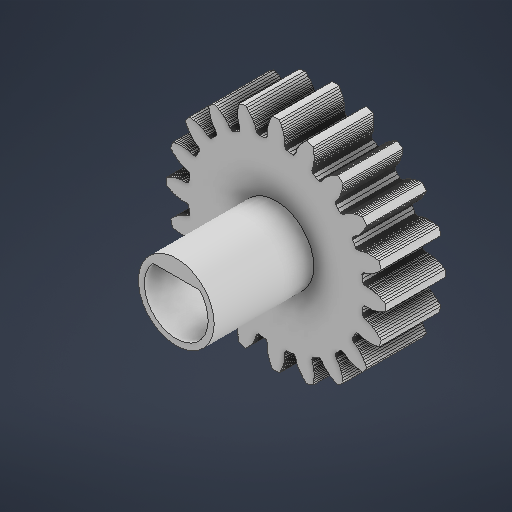
# Autodesk Inventor part: EngranajeMotor
Saved by Autodesk Inventor 2027 (Build 310192060, 192F)
## iProperties
Created: 2026-08-09
Part Number: EngranajeMotor
Material: Generic
Document SubType Name: Modeling
Designer: Administrator
Density: 1 g/cm^3
Appearance: Default
Author: Administrator
Autodesk Inventor part; units mm, degrees
(part 1 of 3)
ref_plane "YZ Plane" through (0, 0, 0) normal (1, 0, 0) x (0, 1, 0)
ref_plane "XZ Plane" through (0, 0, 0) normal (0, 1, 0) x (-1, 0, 0)
ref_plane "XY Plane" through (0, 0, 0) normal (0, 0, 1) x (1, 0, 0)
sketch "Sketch2" plane through (0, 0, 0) normal (0, 0, 1) x (1, 0, 0)
  arc A0 (-1.118, 1) -> (1.118, 1) centre (0, 0) ccw
  arc A1 (-1.118, 1) -> (1.118, 1) centre (0, 0) ccw
  line L0 (0, -0.275) -> (0, 0.275)
  line L1 (-0.275, 0) -> (0.275, 0)
  line L2 (0, -0.275) -> (0, 0.275)
  line L3 (-0.275, 0) -> (0.275, 0)
  line L4 (0, 1) -> (-1.118, 1)
  line L5 (0, 1) -> (1.118, 1)
  line L6 (5.0569, 1.3152) -> (4.9868, 1.2577)
  line L7 (4.9868, 1.2577) -> (4.9194, 1.207)
  line L8 (4.9194, 1.207) -> (4.8581, 1.1647)
  line L9 (4.8581, 1.1647) -> (4.8009, 1.1288)
  line L10 (4.8009, 1.1288) -> (4.75, 1.0997)
  line L11 (4.75, 1.0997) -> (4.7061, 1.0769)
  line L12 (4.7061, 1.0769) -> (4.6364, 1.046)
  line L13 (4.6364, 1.046) -> (4.5924, 1.0307)
  line L14 (4.5924, 1.0307) -> (4.5075, 1.0081)
  line L15 (4.5075, 1.0081) -> (4.4514, 0.9867)
  line L16 (4.4514, 0.9867) -> (4.427, 0.9751)
  line L17 (4.427, 0.9751) -> (4.4051, 0.9628)
  line L18 (4.4051, 0.9628) -> (4.3856, 0.9502)
  line L19 (4.3856, 0.9502) -> (4.3686, 0.9372)
  line L20 (4.3686, 0.9372) -> (4.354, 0.9239)
  line L21 (4.354, 0.9239) -> (4.3419, 0.9105)
  line L22 (4.3419, 0.9105) -> (4.3323, 0.897)
  line L23 (4.3323, 0.897) -> (4.3252, 0.8836)
  line L24 (4.3252, 0.8836) -> (4.3205, 0.8703)
  line L25 (4.3205, 0.8703) -> (4.3182, 0.8572)
  line L26 (4.3182, 0.8572) -> (4.3194, 0.8383)
  line L27 (4.3194, 0.8383) -> (4.3458, 0.6883)
  line L28 (4.3458, 0.6883) -> (4.3671, 0.5375)
  line L29 (4.3671, 0.5375) -> (4.3718, 0.5191)
  line L30 (4.3718, 0.5191) -> (4.378, 0.5074)
  line L31 (4.378, 0.5074) -> (4.3865, 0.4962)
  line L32 (4.3865, 0.4962) -> (4.3975, 0.4856)
  line L33 (4.3975, 0.4856) -> (4.4108, 0.4758)
  line L34 (4.4108, 0.4758) -> (4.4264, 0.4668)
  line L35 (4.4264, 0.4668) -> (4.4444, 0.4587)
  line L36 (4.4444, 0.4587) -> (4.4646, 0.4516)
  line L37 (4.4646, 0.4516) -> (4.487, 0.4455)
  line L38 (4.487, 0.4455) -> (4.5117, 0.4407)
  line L39 (4.5117, 0.4407) -> (4.5385, 0.4371)
  line L40 (4.5385, 0.4371) -> (4.5984, 0.4341)
  line L41 (4.5984, 0.4341) -> (4.6862, 0.4388)
  line L42 (4.6862, 0.4388) -> (4.7327, 0.438)
  line L43 (4.7327, 0.438) -> (4.8085, 0.43)
  line L44 (4.8085, 0.43) -> (4.8574, 0.422)
  line L45 (4.8574, 0.422) -> (4.9147, 0.41)
  line L46 (4.9147, 0.41) -> (4.9802, 0.3935)
  line L47 (4.9802, 0.3935) -> (5.0516, 0.3723)
  line L48 (5.0516, 0.3723) -> (5.1313, 0.3449)
  line L49 (5.1313, 0.3449) -> (5.2159, 0.3118)
  line L50 (5.2159, 0.3118) -> (5.3081, 0.2712)
  line L51 (5.3081, 0.2712) -> (5.4053, 0.2235)
  line L52 (5.4053, 0.2235) -> (5.4973, 0.1736)
  arc A2 (5.4973, -0.1736) -> (5.4973, 0.1736) centre (0, 0) ccw
  line L53 (5.4973, -0.1736) -> (5.4053, -0.2235)
  line L54 (5.4053, -0.2235) -> (5.3081, -0.2712)
  line L55 (5.3081, -0.2712) -> (5.2159, -0.3118)
  line L56 (5.2159, -0.3118) -> (5.1313, -0.3449)
  line L57 (5.1313, -0.3449) -> (5.0516, -0.3723)
  line L58 (5.0516, -0.3723) -> (4.9802, -0.3935)
  line L59 (4.9802, -0.3935) -> (4.9147, -0.41)
  line L60 (4.9147, -0.41) -> (4.8574, -0.422)
  line L61 (4.8574, -0.422) -> (4.8085, -0.43)
  line L62 (4.8085, -0.43) -> (4.7327, -0.438)
  line L63 (4.7327, -0.438) -> (4.6862, -0.4388)
  line L64 (4.6862, -0.4388) -> (4.5984, -0.4341)
  line L65 (4.5984, -0.4341) -> (4.5385, -0.4371)
  line L66 (4.5385, -0.4371) -> (4.5117, -0.4407)
  line L67 (4.5117, -0.4407) -> (4.487, -0.4455)
  line L68 (4.487, -0.4455) -> (4.4646, -0.4516)
  line L69 (4.4646, -0.4516) -> (4.4444, -0.4587)
  line L70 (4.4444, -0.4587) -> (4.4264, -0.4668)
  line L71 (4.4264, -0.4668) -> (4.4108, -0.4758)
  line L72 (4.4108, -0.4758) -> (4.3975, -0.4856)
  line L73 (4.3975, -0.4856) -> (4.3865, -0.4962)
  line L74 (4.3865, -0.4962) -> (4.378, -0.5074)
  line L75 (4.378, -0.5074) -> (4.3718, -0.5191)
  line L76 (4.3718, -0.5191) -> (4.3671, -0.5375)
  line L77 (4.3671, -0.5375) -> (4.3458, -0.6883)
  line L78 (4.3458, -0.6883) -> (4.3194, -0.8383)
  line L79 (4.3194, -0.8383) -> (4.3182, -0.8572)
  line L80 (4.3182, -0.8572) -> (4.3205, -0.8703)
  line L81 (4.3205, -0.8703) -> (4.3252, -0.8836)
  line L82 (4.3252, -0.8836) -> (4.3323, -0.897)
  line L83 (4.3323, -0.897) -> (4.3419, -0.9105)
  line L84 (4.3419, -0.9105) -> (4.354, -0.9239)
  line L85 (4.354, -0.9239) -> (4.3686, -0.9372)
  line L86 (4.3686, -0.9372) -> (4.3856, -0.9502)
  line L87 (4.3856, -0.9502) -> (4.4051, -0.9628)
  line L88 (4.4051, -0.9628) -> (4.427, -0.9751)
  line L89 (4.427, -0.9751) -> (4.4514, -0.9867)
  line L90 (4.4514, -0.9867) -> (4.5075, -1.0081)
  line L91 (4.5075, -1.0081) -> (4.5924, -1.0307)
  line L92 (4.5924, -1.0307) -> (4.6364, -1.046)
  line L93 (4.6364, -1.046) -> (4.7061, -1.0769)
  line L94 (4.7061, -1.0769) -> (4.75, -1.0997)
  line L95 (4.75, -1.0997) -> (4.8009, -1.1288)
  line L96 (4.8009, -1.1288) -> (4.8581, -1.1647)
  line L97 (4.8581, -1.1647) -> (4.9194, -1.207)
  line L98 (4.9194, -1.207) -> (4.9868, -1.2577)
  line L99 (4.9868, -1.2577) -> (5.0569, -1.3152)
  line L100 (5.0569, -1.3152) -> (5.1322, -1.3823)
  line L101 (5.1322, -1.3823) -> (5.2098, -1.4578)
  line L102 (5.2098, -1.4578) -> (5.2818, -1.5336)
  arc A3 (5.1745, -1.8639) -> (5.2818, -1.5336) centre (0, 0) ccw
  line L103 (5.1745, -1.8639) -> (5.0717, -1.8829)
  line L104 (5.0717, -1.8829) -> (4.9645, -1.8983)
  line L105 (4.9645, -1.8983) -> (4.8642, -1.9084)
  line L106 (4.8642, -1.9084) -> (4.7736, -1.9137)
  line L107 (4.7736, -1.9137) -> (4.6893, -1.9151)
  line L108 (4.6893, -1.9151) -> (4.6149, -1.9132)
  line L109 (4.6149, -1.9132) -> (4.5475, -1.9087)
  line L110 (4.5475, -1.9087) -> (4.4892, -1.9023)
  line L111 (4.4892, -1.9023) -> (4.4403, -1.8949)
  line L112 (4.4403, -1.8949) -> (4.3657, -1.879)
  line L113 (4.3657, -1.879) -> (4.3212, -1.8655)
  line L114 (4.3212, -1.8655) -> (4.2391, -1.8339)
  line L115 (4.2391, -1.8339) -> (4.1813, -1.8182)
  line L116 (4.1813, -1.8182) -> (4.1547, -1.8133)
  line L117 (4.1547, -1.8133) -> (4.1297, -1.8103)
  line L118 (4.1297, -1.8103) -> (4.1065, -1.8091)
  line L119 (4.1065, -1.8091) -> (4.0851, -1.8096)
  line L120 (4.0851, -1.8096) -> (4.0655, -1.8118)
  line L121 (4.0655, -1.8118) -> (4.0479, -1.8155)
  line L122 (4.0479, -1.8155) -> (4.0322, -1.8208)
  line L123 (4.0322, -1.8208) -> (4.0185, -1.8274)
  line L124 (4.0185, -1.8274) -> (4.0069, -1.8354)
  line L125 (4.0069, -1.8354) -> (3.9974, -1.8447)
  line L126 (3.9974, -1.8447) -> (3.9872, -1.8607)
  line L127 (3.9872, -1.8607) -> (3.9204, -1.9976)
  line L128 (3.9204, -1.9976) -> (3.8489, -2.1321)
  line L129 (3.8489, -2.1321) -> (3.842, -2.1497)
  line L130 (3.842, -2.1497) -> (3.8401, -2.1628)
  line L131 (3.8401, -2.1628) -> (3.8404, -2.1769)
  line L132 (3.8404, -2.1769) -> (3.8431, -2.1919)
  line L133 (3.8431, -2.1919) -> (3.8481, -2.2077)
  line L134 (3.8481, -2.2077) -> (3.8554, -2.2242)
  line L135 (3.8554, -2.2242) -> (3.8652, -2.2413)
  line L136 (3.8652, -2.2413) -> (3.8773, -2.2589)
  line L137 (3.8773, -2.2589) -> (3.892, -2.277)
  line L138 (3.892, -2.277) -> (3.9091, -2.2954)
  line L139 (3.9091, -2.2954) -> (3.9286, -2.314)
  line L140 (3.9286, -2.314) -> (3.9753, -2.3516)
  line L141 (3.9753, -2.3516) -> (4.0491, -2.3994)
  line L142 (4.0491, -2.3994) -> (4.0862, -2.4275)
  line L143 (4.0862, -2.4275) -> (4.1429, -2.4785)
  line L144 (4.1429, -2.4785) -> (4.1777, -2.5137)
  line L145 (4.1777, -2.5137) -> (4.2171, -2.5571)
  line L146 (4.2171, -2.5571) -> (4.2604, -2.609)
  line L147 (4.2604, -2.609) -> (4.3057, -2.6681)
  line L148 (4.3057, -2.6681) -> (4.3541, -2.7371)
  line L149 (4.3541, -2.7371) -> (4.403, -2.8135)
  line L150 (4.403, -2.8135) -> (4.4538, -2.9006)
  line L151 (4.4538, -2.9006) -> (4.5044, -2.9964)
  line L152 (4.5044, -2.9964) -> (4.5494, -3.0907)
  arc A4 (4.3453, -3.3717) -> (4.5494, -3.0907) centre (0, 0) ccw
  line L153 (4.3453, -3.3717) -> (4.2416, -3.358)
  line L154 (4.2416, -3.358) -> (4.1349, -3.3395)
  line L155 (4.1349, -3.3395) -> (4.0364, -3.3181)
  line L156 (4.0364, -3.3181) -> (3.9486, -3.2952)
  line L157 (3.9486, -3.2952) -> (3.868, -3.2704)
  line L158 (3.868, -3.2704) -> (3.7978, -3.2457)
  line L159 (3.7978, -3.2457) -> (3.7351, -3.2205)
  line L160 (3.7351, -3.2205) -> (3.6817, -3.1965)
  line L161 (3.6817, -3.1965) -> (3.6374, -3.1743)
  line L162 (3.6374, -3.1743) -> (3.5714, -3.1361)
  line L163 (3.5714, -3.1361) -> (3.5332, -3.1095)
  line L164 (3.5332, -3.1095) -> (3.465, -3.0541)
  line L165 (3.465, -3.0541) -> (3.4148, -3.0213)
  line L166 (3.4148, -3.0213) -> (3.391, -3.0084)
  line L167 (3.391, -3.0084) -> (3.3682, -2.9979)
  line L168 (3.3682, -2.9979) -> (3.3465, -2.9895)
  line L169 (3.3465, -2.9895) -> (3.326, -2.9834)
  line L170 (3.326, -2.9834) -> (3.3067, -2.9794)
  line L171 (3.3067, -2.9794) -> (3.2887, -2.9775)
  line L172 (3.2887, -2.9775) -> (3.2722, -2.9777)
  line L173 (3.2722, -2.9777) -> (3.2571, -2.9798)
  line L174 (3.2571, -2.9798) -> (3.2436, -2.9838)
  line L175 (3.2436, -2.9838) -> (3.2317, -2.9896)
  line L176 (3.2317, -2.9896) -> (3.2171, -3.0017)
  line L177 (3.2171, -3.0017) -> (3.1113, -3.1113)
  line L178 (3.1113, -3.1113) -> (3.0017, -3.2171)
  line L179 (3.0017, -3.2171) -> (2.9896, -3.2317)
  line L180 (2.9896, -3.2317) -> (2.9838, -3.2436)
  line L181 (2.9838, -3.2436) -> (2.9798, -3.2571)
  line L182 (2.9798, -3.2571) -> (2.9777, -3.2722)
  line L183 (2.9777, -3.2722) -> (2.9775, -3.2887)
  line L184 (2.9775, -3.2887) -> (2.9794, -3.3067)
  line L185 (2.9794, -3.3067) -> (2.9834, -3.326)
  line L186 (2.9834, -3.326) -> (2.9895, -3.3465)
  line L187 (2.9895, -3.3465) -> (2.9979, -3.3682)
  line L188 (2.9979, -3.3682) -> (3.0084, -3.391)
  line L189 (3.0084, -3.391) -> (3.0213, -3.4148)
  line L190 (3.0213, -3.4148) -> (3.0541, -3.465)
  line L191 (3.0541, -3.465) -> (3.1095, -3.5332)
  line L192 (3.1095, -3.5332) -> (3.1361, -3.5714)
  line L193 (3.1361, -3.5714) -> (3.1743, -3.6374)
  line L194 (3.1743, -3.6374) -> (3.1965, -3.6817)
  line L195 (3.1965, -3.6817) -> (3.2205, -3.7351)
  line L196 (3.2205, -3.7351) -> (3.2457, -3.7978)
  line L197 (3.2457, -3.7978) -> (3.2704, -3.868)
  line L198 (3.2704, -3.868) -> (3.2952, -3.9486)
  line L199 (3.2952, -3.9486) -> (3.3181, -4.0364)
  line L200 (3.3181, -4.0364) -> (3.3395, -4.1349)
  line L201 (3.3395, -4.1349) -> (3.358, -4.2416)
  line L202 (3.358, -4.2416) -> (3.3717, -4.3453)
  arc A5 (3.0907, -4.5494) -> (3.3717, -4.3453) centre (0, 0) ccw
  line L203 (3.0907, -4.5494) -> (2.9964, -4.5044)
  line L204 (2.9964, -4.5044) -> (2.9006, -4.4538)
  line L205 (2.9006, -4.4538) -> (2.8135, -4.403)
  line L206 (2.8135, -4.403) -> (2.7371, -4.3541)
  line L207 (2.7371, -4.3541) -> (2.6681, -4.3057)
  line L208 (2.6681, -4.3057) -> (2.609, -4.2604)
  line L209 (2.609, -4.2604) -> (2.5571, -4.2171)
  line L210 (2.5571, -4.2171) -> (2.5137, -4.1777)
  line L211 (2.5137, -4.1777) -> (2.4785, -4.1429)
  line L212 (2.4785, -4.1429) -> (2.4275, -4.0862)
  line L213 (2.4275, -4.0862) -> (2.3994, -4.0491)
  line L214 (2.3994, -4.0491) -> (2.3516, -3.9753)
  line L215 (2.3516, -3.9753) -> (2.314, -3.9286)
  line L216 (2.314, -3.9286) -> (2.2954, -3.9091)
  line L217 (2.2954, -3.9091) -> (2.277, -3.892)
  line L218 (2.277, -3.892) -> (2.2589, -3.8773)
  line L219 (2.2589, -3.8773) -> (2.2413, -3.8652)
  line L220 (2.2413, -3.8652) -> (2.2242, -3.8554)
  line L221 (2.2242, -3.8554) -> (2.2077, -3.8481)
  line L222 (2.2077, -3.8481) -> (2.1919, -3.8431)
  line L223 (2.1919, -3.8431) -> (2.1769, -3.8404)
  line L224 (2.1769, -3.8404) -> (2.1628, -3.8401)
  line L225 (2.1628, -3.8401) -> (2.1497, -3.842)
  line L226 (2.1497, -3.842) -> (2.1321, -3.8489)
  line L227 (2.1321, -3.8489) -> (1.9976, -3.9204)
  line L228 (1.9976, -3.9204) -> (1.8607, -3.9872)
  line L229 (1.8607, -3.9872) -> (1.8447, -3.9974)
  line L230 (1.8447, -3.9974) -> (1.8354, -4.0069)
  line L231 (1.8354, -4.0069) -> (1.8274, -4.0185)
  line L232 (1.8274, -4.0185) -> (1.8208, -4.0322)
  line L233 (1.8208, -4.0322) -> (1.8155, -4.0479)
  line L234 (1.8155, -4.0479) -> (1.8118, -4.0655)
  line L235 (1.8118, -4.0655) -> (1.8096, -4.0851)
  line L236 (1.8096, -4.0851) -> (1.8091, -4.1065)
  line L237 (1.8091, -4.1065) -> (1.8103, -4.1297)
  line L238 (1.8103, -4.1297) -> (1.8133, -4.1547)
  line L239 (1.8133, -4.1547) -> (1.8182, -4.1813)
  line L240 (1.8182, -4.1813) -> (1.8339, -4.2391)
  line L241 (1.8339, -4.2391) -> (1.8655, -4.3212)
  line L242 (1.8655, -4.3212) -> (1.879, -4.3657)
  line L243 (1.879, -4.3657) -> (1.8949, -4.4403)
  line L244 (1.8949, -4.4403) -> (1.9023, -4.4892)
  line L245 (1.9023, -4.4892) -> (1.9087, -4.5475)
  line L246 (1.9087, -4.5475) -> (1.9132, -4.6149)
  line L247 (1.9132, -4.6149) -> (1.9151, -4.6893)
  line L248 (1.9151, -4.6893) -> (1.9137, -4.7736)
  line L249 (1.9137, -4.7736) -> (1.9084, -4.8642)
  line L250 (1.9084, -4.8642) -> (1.8983, -4.9645)
  line L251 (1.8983, -4.9645) -> (1.8829, -5.0717)
  line L252 (1.8829, -5.0717) -> (1.8639, -5.1745)
  arc A6 (1.5336, -5.2818) -> (1.8639, -5.1745) centre (0, 0) ccw
  line L253 (1.5336, -5.2818) -> (1.4578, -5.2098)
  line L254 (1.4578, -5.2098) -> (1.3823, -5.1322)
  line L255 (1.3823, -5.1322) -> (1.3152, -5.0569)
  line L256 (1.3152, -5.0569) -> (1.2577, -4.9868)
  line L257 (1.2577, -4.9868) -> (1.207, -4.9194)
  line L258 (1.207, -4.9194) -> (1.1647, -4.8581)
  line L259 (1.1647, -4.8581) -> (1.1288, -4.8009)
  line L260 (1.1288, -4.8009) -> (1.0997, -4.75)
  line L261 (1.0997, -4.75) -> (1.0769, -4.7061)
  line L262 (1.0769, -4.7061) -> (1.046, -4.6364)
  line L263 (1.046, -4.6364) -> (1.0307, -4.5924)
  line L264 (1.0307, -4.5924) -> (1.0081, -4.5075)
  line L265 (1.0081, -4.5075) -> (0.9867, -4.4514)
  line L266 (0.9867, -4.4514) -> (0.9751, -4.427)
  line L267 (0.9751, -4.427) -> (0.9628, -4.4051)
  line L268 (0.9628, -4.4051) -> (0.9502, -4.3856)
  line L269 (0.9502, -4.3856) -> (0.9372, -4.3686)
  line L270 (0.9372, -4.3686) -> (0.9239, -4.354)
  line L271 (0.9239, -4.354) -> (0.9105, -4.3419)
  line L272 (0.9105, -4.3419) -> (0.897, -4.3323)
  line L273 (0.897, -4.3323) -> (0.8836, -4.3252)
  line L274 (0.8836, -4.3252) -> (0.8703, -4.3205)
  line L275 (0.8703, -4.3205) -> (0.8572, -4.3182)
  line L276 (0.8572, -4.3182) -> (0.8383, -4.3194)
  line L277 (0.8383, -4.3194) -> (0.6883, -4.3458)
  line L278 (0.6883, -4.3458) -> (0.5375, -4.3671)
  line L279 (0.5375, -4.3671) -> (0.5191, -4.3718)
  line L280 (0.5191, -4.3718) -> (0.5074, -4.378)
  line L281 (0.5074, -4.378) -> (0.4962, -4.3865)
  line L282 (0.4962, -4.3865) -> (0.4856, -4.3975)
  line L283 (0.4856, -4.3975) -> (0.4758, -4.4108)
  line L284 (0.4758, -4.4108) -> (0.4668, -4.4264)
  line L285 (0.4668, -4.4264) -> (0.4587, -4.4444)
  line L286 (0.4587, -4.4444) -> (0.4516, -4.4646)
  line L287 (0.4516, -4.4646) -> (0.4455, -4.487)
  line L288 (0.4455, -4.487) -> (0.4407, -4.5117)
  line L289 (0.4407, -4.5117) -> (0.4371, -4.5385)
  line L290 (0.4371, -4.5385) -> (0.4341, -4.5984)
  line L291 (0.4341, -4.5984) -> (0.4388, -4.6862)
  line L292 (0.4388, -4.6862) -> (0.438, -4.7327)
  line L293 (0.438, -4.7327) -> (0.43, -4.8085)
  line L294 (0.43, -4.8085) -> (0.422, -4.8574)
  line L295 (0.422, -4.8574) -> (0.41, -4.9147)
  line L296 (0.41, -4.9147) -> (0.3935, -4.9802)
  line L297 (0.3935, -4.9802) -> (0.3723, -5.0516)
  line L298 (0.3723, -5.0516) -> (0.3449, -5.1313)
  line L299 (0.3449, -5.1313) -> (0.3118, -5.2159)
  line L300 (0.3118, -5.2159) -> (0.2712, -5.3081)
  line L301 (0.2712, -5.3081) -> (0.2235, -5.4053)
  line L302 (0.2235, -5.4053) -> (0.1736, -5.4973)
  arc A7 (-0.1736, -5.4973) -> (0.1736, -5.4973) centre (0, 0) ccw
  line L303 (-0.1736, -5.4973) -> (-0.2235, -5.4053)
  line L304 (-0.2235, -5.4053) -> (-0.2712, -5.3081)
  line L305 (-0.2712, -5.3081) -> (-0.3118, -5.2159)
  line L306 (-0.3118, -5.2159) -> (-0.3449, -5.1313)
  line L307 (-0.3449, -5.1313) -> (-0.3723, -5.0516)
  line L308 (-0.3723, -5.0516) -> (-0.3935, -4.9802)
  line L309 (-0.3935, -4.9802) -> (-0.41, -4.9147)
  line L310 (-0.41, -4.9147) -> (-0.422, -4.8574)
  line L311 (-0.422, -4.8574) -> (-0.43, -4.8085)
  line L312 (-0.43, -4.8085) -> (-0.438, -4.7327)
  line L313 (-0.438, -4.7327) -> (-0.4388, -4.6862)
  line L314 (-0.4388, -4.6862) -> (-0.4341, -4.5984)
  line L315 (-0.4341, -4.5984) -> (-0.4371, -4.5385)
  line L316 (-0.4371, -4.5385) -> (-0.4407, -4.5117)
  line L317 (-0.4407, -4.5117) -> (-0.4455, -4.487)
  line L318 (-0.4455, -4.487) -> (-0.4516, -4.4646)
  line L319 (-0.4516, -4.4646) -> (-0.4587, -4.4444)
  line L320 (-0.4587, -4.4444) -> (-0.4668, -4.4264)
  line L321 (-0.4668, -4.4264) -> (-0.4758, -4.4108)
  line L322 (-0.4758, -4.4108) -> (-0.4856, -4.3975)
  line L323 (-0.4856, -4.3975) -> (-0.4962, -4.3865)
  line L324 (-0.4962, -4.3865) -> (-0.5074, -4.378)
  line L325 (-0.5074, -4.378) -> (-0.5191, -4.3718)
  line L326 (-0.5191, -4.3718) -> (-0.5375, -4.3671)
  line L327 (-0.5375, -4.3671) -> (-0.6883, -4.3458)
  line L328 (-0.6883, -4.3458) -> (-0.8383, -4.3194)
  line L329 (-0.8383, -4.3194) -> (-0.8572, -4.3182)
  line L330 (-0.8572, -4.3182) -> (-0.8703, -4.3205)
  line L331 (-0.8703, -4.3205) -> (-0.8836, -4.3252)
  line L332 (-0.8836, -4.3252) -> (-0.897, -4.3323)
  line L333 (-0.897, -4.3323) -> (-0.9105, -4.3419)
  line L334 (-0.9105, -4.3419) -> (-0.9239, -4.354)
  line L335 (-0.9239, -4.354) -> (-0.9372, -4.3686)
  line L336 (-0.9372, -4.3686) -> (-0.9502, -4.3856)
  line L337 (-0.9502, -4.3856) -> (-0.9628, -4.4051)
  line L338 (-0.9628, -4.4051) -> (-0.9751, -4.427)
  line L339 (-0.9751, -4.427) -> (-0.9867, -4.4514)
  line L340 (-0.9867, -4.4514) -> (-1.0081, -4.5075)
  line L341 (-1.0081, -4.5075) -> (-1.0307, -4.5924)
  line L342 (-1.0307, -4.5924) -> (-1.046, -4.6364)
  line L343 (-1.046, -4.6364) -> (-1.0769, -4.7061)
  line L344 (-1.0769, -4.7061) -> (-1.0997, -4.75)
  line L345 (-1.0997, -4.75) -> (-1.1288, -4.8009)
  line L346 (-1.1288, -4.8009) -> (-1.1647, -4.8581)
  line L347 (-1.1647, -4.8581) -> (-1.207, -4.9194)
  line L348 (-1.207, -4.9194) -> (-1.2577, -4.9868)
  line L349 (-1.2577, -4.9868) -> (-1.3152, -5.0569)
  line L350 (-1.3152, -5.0569) -> (-1.3823, -5.1322)
  line L351 (-1.3823, -5.1322) -> (-1.4578, -5.2098)
  line L352 (-1.4578, -5.2098) -> (-1.5336, -5.2818)
  arc A8 (-1.8639, -5.1745) -> (-1.5336, -5.2818) centre (0, 0) ccw
  line L353 (-1.8639, -5.1745) -> (-1.8829, -5.0717)
  line L354 (-1.8829, -5.0717) -> (-1.8983, -4.9645)
  line L355 (-1.8983, -4.9645) -> (-1.9084, -4.8642)
  line L356 (-1.9084, -4.8642) -> (-1.9137, -4.7736)
  line L357 (-1.9137, -4.7736) -> (-1.9151, -4.6893)
  line L358 (-1.9151, -4.6893) -> (-1.9132, -4.6149)
  line L359 (-1.9132, -4.6149) -> (-1.9087, -4.5475)
  line L360 (-1.9087, -4.5475) -> (-1.9023, -4.4892)
  line L361 (-1.9023, -4.4892) -> (-1.8949, -4.4403)
  line L362 (-1.8949, -4.4403) -> (-1.879, -4.3657)
  line L363 (-1.879, -4.3657) -> (-1.8655, -4.3212)
  line L364 (-1.8655, -4.3212) -> (-1.8339, -4.2391)
  line L365 (-1.8339, -4.2391) -> (-1.8182, -4.1813)
  line L366 (-1.8182, -4.1813) -> (-1.8133, -4.1547)
  line L367 (-1.8133, -4.1547) -> (-1.8103, -4.1297)
  line L368 (-1.8103, -4.1297) -> (-1.8091, -4.1065)
  line L369 (-1.8091, -4.1065) -> (-1.8096, -4.0851)
  line L370 (-1.8096, -4.0851) -> (-1.8118, -4.0655)
  line L371 (-1.8118, -4.0655) -> (-1.8155, -4.0479)
  line L372 (-1.8155, -4.0479) -> (-1.8208, -4.0322)
  line L373 (-1.8208, -4.0322) -> (-1.8274, -4.0185)
  line L374 (-1.8274, -4.0185) -> (-1.8354, -4.0069)
  line L375 (-1.8354, -4.0069) -> (-1.8447, -3.9974)
  line L376 (-1.8447, -3.9974) -> (-1.8607, -3.9872)
  line L377 (-1.8607, -3.9872) -> (-1.9976, -3.9204)
  line L378 (-1.9976, -3.9204) -> (-2.1321, -3.8489)
  line L379 (-2.1321, -3.8489) -> (-2.1497, -3.842)
  line L380 (-2.1497, -3.842) -> (-2.1628, -3.8401)
  line L381 (-2.1628, -3.8401) -> (-2.1769, -3.8404)
  line L382 (-2.1769, -3.8404) -> (-2.1919, -3.8431)
  line L383 (-2.1919, -3.8431) -> (-2.2077, -3.8481)
  line L384 (-2.2077, -3.8481) -> (-2.2242, -3.8554)
  line L385 (-2.2242, -3.8554) -> (-2.2413, -3.8652)
  line L386 (-2.2413, -3.8652) -> (-2.2589, -3.8773)
  line L387 (-2.2589, -3.8773) -> (-2.277, -3.892)
  line L388 (-2.277, -3.892) -> (-2.2954, -3.9091)
  line L389 (-2.2954, -3.9091) -> (-2.314, -3.9286)
  line L390 (-2.314, -3.9286) -> (-2.3516, -3.9753)
  line L391 (-2.3516, -3.9753) -> (-2.3994, -4.0491)
  line L392 (-2.3994, -4.0491) -> (-2.4275, -4.0862)
  line L393 (-2.4275, -4.0862) -> (-2.4785, -4.1429)
  line L394 (-2.4785, -4.1429) -> (-2.5137, -4.1777)
  line L395 (-2.5137, -4.1777) -> (-2.5571, -4.2171)
  line L396 (-2.5571, -4.2171) -> (-2.609, -4.2604)
  line L397 (-2.609, -4.2604) -> (-2.6681, -4.3057)
  line L398 (-2.6681, -4.3057) -> (-2.7371, -4.3541)
  line L399 (-2.7371, -4.3541) -> (-2.8135, -4.403)
  line L400 (-2.8135, -4.403) -> (-2.9006, -4.4538)
  line L401 (-2.9006, -4.4538) -> (-2.9964, -4.5044)
  line L402 (-2.9964, -4.5044) -> (-3.0907, -4.5494)
  arc A9 (-3.3717, -4.3453) -> (-3.0907, -4.5494) centre (0, 0) ccw
  line L403 (-3.3717, -4.3453) -> (-3.358, -4.2416)
  line L404 (-3.358, -4.2416) -> (-3.3395, -4.1349)
  line L405 (-3.3395, -4.1349) -> (-3.3181, -4.0364)
  line L406 (-3.3181, -4.0364) -> (-3.2952, -3.9486)
  line L407 (-3.2952, -3.9486) -> (-3.2704, -3.868)
  line L408 (-3.2704, -3.868) -> (-3.2457, -3.7978)
  line L409 (-3.2457, -3.7978) -> (-3.2205, -3.7351)
  line L410 (-3.2205, -3.7351) -> (-3.1965, -3.6817)
  line L411 (-3.1965, -3.6817) -> (-3.1743, -3.6374)
  line L412 (-3.1743, -3.6374) -> (-3.1361, -3.5714)
  line L413 (-3.1361, -3.5714) -> (-3.1095, -3.5332)
  line L414 (-3.1095, -3.5332) -> (-3.0541, -3.465)
  line L415 (-3.0541, -3.465) -> (-3.0213, -3.4148)
  line L416 (-3.0213, -3.4148) -> (-3.0084, -3.391)
  line L417 (-3.0084, -3.391) -> (-2.9979, -3.3682)
  line L418 (-2.9979, -3.3682) -> (-2.9895, -3.3465)
  line L419 (-2.9895, -3.3465) -> (-2.9834, -3.326)
  line L420 (-2.9834, -3.326) -> (-2.9794, -3.3067)
  line L421 (-2.9794, -3.3067) -> (-2.9775, -3.2887)
  line L422 (-2.9775, -3.2887) -> (-2.9777, -3.2722)
  line L423 (-2.9777, -3.2722) -> (-2.9798, -3.2571)
  line L424 (-2.9798, -3.2571) -> (-2.9838, -3.2436)
  line L425 (-2.9838, -3.2436) -> (-2.9896, -3.2317)
  line L426 (-2.9896, -3.2317) -> (-3.0017, -3.2171)
  line L427 (-3.0017, -3.2171) -> (-3.1113, -3.1113)
  line L428 (-3.1113, -3.1113) -> (-3.2171, -3.0017)
  line L429 (-3.2171, -3.0017) -> (-3.2317, -2.9896)
  line L430 (-3.2317, -2.9896) -> (-3.2436, -2.9838)
  line L431 (-3.2436, -2.9838) -> (-3.2571, -2.9798)
  line L432 (-3.2571, -2.9798) -> (-3.2722, -2.9777)
  line L433 (-3.2722, -2.9777) -> (-3.2887, -2.9775)
  line L434 (-3.2887, -2.9775) -> (-3.3067, -2.9794)
  line L435 (-3.3067, -2.9794) -> (-3.326, -2.9834)
  line L436 (-3.326, -2.9834) -> (-3.3465, -2.9895)
  line L437 (-3.3465, -2.9895) -> (-3.3682, -2.9979)
  line L438 (-3.3682, -2.9979) -> (-3.391, -3.0084)
  line L439 (-3.391, -3.0084) -> (-3.4148, -3.0213)
  line L440 (-3.4148, -3.0213) -> (-3.465, -3.0541)
  line L441 (-3.465, -3.0541) -> (-3.5332, -3.1095)
  line L442 (-3.5332, -3.1095) -> (-3.5714, -3.1361)
  line L443 (-3.5714, -3.1361) -> (-3.6374, -3.1743)
  line L444 (-3.6374, -3.1743) -> (-3.6817, -3.1965)
  line L445 (-3.6817, -3.1965) -> (-3.7351, -3.2205)
  line L446 (-3.7351, -3.2205) -> (-3.7978, -3.2457)
  line L447 (-3.7978, -3.2457) -> (-3.868, -3.2704)
  line L448 (-3.868, -3.2704) -> (-3.9486, -3.2952)
  line L449 (-3.9486, -3.2952) -> (-4.0364, -3.3181)
  line L450 (-4.0364, -3.3181) -> (-4.1349, -3.3395)
  line L451 (-4.1349, -3.3395) -> (-4.2416, -3.358)
  line L452 (-4.2416, -3.358) -> (-4.3453, -3.3717)
  arc A10 (-4.5494, -3.0907) -> (-4.3453, -3.3717) centre (0, 0) ccw
  line L453 (-4.5494, -3.0907) -> (-4.5044, -2.9964)
  line L454 (-4.5044, -2.9964) -> (-4.4538, -2.9006)
  line L455 (-4.4538, -2.9006) -> (-4.403, -2.8135)
  line L456 (-4.403, -2.8135) -> (-4.3541, -2.7371)
  line L457 (-4.3541, -2.7371) -> (-4.3057, -2.6681)
  line L458 (-4.3057, -2.6681) -> (-4.2604, -2.609)
  line L459 (-4.2604, -2.609) -> (-4.2171, -2.5571)
  line L460 (-4.2171, -2.5571) -> (-4.1777, -2.5137)
  line L461 (-4.1777, -2.5137) -> (-4.1429, -2.4785)
  line L462 (-4.1429, -2.4785) -> (-4.0862, -2.4275)
  line L463 (-4.0862, -2.4275) -> (-4.0491, -2.3994)
  line L464 (-4.0491, -2.3994) -> (-3.9753, -2.3516)
  line L465 (-3.9753, -2.3516) -> (-3.9286, -2.314)
  line L466 (-3.9286, -2.314) -> (-3.9091, -2.2954)
  line L467 (-3.9091, -2.2954) -> (-3.892, -2.277)
  line L468 (-3.892, -2.277) -> (-3.8773, -2.2589)
  line L469 (-3.8773, -2.2589) -> (-3.8652, -2.2413)
  line L470 (-3.8652, -2.2413) -> (-3.8554, -2.2242)
  line L471 (-3.8554, -2.2242) -> (-3.8481, -2.2077)
  line L472 (-3.8481, -2.2077) -> (-3.8431, -2.1919)
  line L473 (-3.8431, -2.1919) -> (-3.8404, -2.1769)
  line L474 (-3.8404, -2.1769) -> (-3.8401, -2.1628)
  line L475 (-3.8401, -2.1628) -> (-3.842, -2.1497)
  line L476 (-3.842, -2.1497) -> (-3.8489, -2.1321)
  line L477 (-3.8489, -2.1321) -> (-3.9204, -1.9976)
  line L478 (-3.9204, -1.9976) -> (-3.9872, -1.8607)
  line L479 (-3.9872, -1.8607) -> (-3.9974, -1.8447)
  line L480 (-3.9974, -1.8447) -> (-4.0069, -1.8354)
  line L481 (-4.0069, -1.8354) -> (-4.0185, -1.8274)
  line L482 (-4.0185, -1.8274) -> (-4.0322, -1.8208)
  line L483 (-4.0322, -1.8208) -> (-4.0479, -1.8155)
  line L484 (-4.0479, -1.8155) -> (-4.0655, -1.8118)
  line L485 (-4.0655, -1.8118) -> (-4.0851, -1.8096)
  line L486 (-4.0851, -1.8096) -> (-4.1065, -1.8091)
  line L487 (-4.1065, -1.8091) -> (-4.1297, -1.8103)
  line L488 (-4.1297, -1.8103) -> (-4.1547, -1.8133)
  line L489 (-4.1547, -1.8133) -> (-4.1813, -1.8182)
  line L490 (-4.1813, -1.8182) -> (-4.2391, -1.8339)
  line L491 (-4.2391, -1.8339) -> (-4.3212, -1.8655)
  line L492 (-4.3212, -1.8655) -> (-4.3657, -1.879)
  line L493 (-4.3657, -1.879) -> (-4.4403, -1.8949)
  line L494 (-4.4403, -1.8949) -> (-4.4892, -1.9023)
  line L495 (-4.4892, -1.9023) -> (-4.5475, -1.9087)
  line L496 (-4.5475, -1.9087) -> (-4.6149, -1.9132)
  line L497 (-4.6149, -1.9132) -> (-4.6893, -1.9151)
  line L498 (-4.6893, -1.9151) -> (-4.7736, -1.9137)
  line L499 (-4.7736, -1.9137) -> (-4.8642, -1.9084)
  line L500 (-4.8642, -1.9084) -> (-4.9645, -1.8983)
  line L501 (-4.9645, -1.8983) -> (-5.0717, -1.8829)
  line L502 (-5.0717, -1.8829) -> (-5.1745, -1.8639)
  arc A11 (-5.2818, -1.5336) -> (-5.1745, -1.8639) centre (0, 0) ccw
  line L503 (-5.2818, -1.5336) -> (-5.2098, -1.4578)
  line L504 (-5.2098, -1.4578) -> (-5.1322, -1.3823)
  line L505 (-5.1322, -1.3823) -> (-5.0569, -1.3152)
  line L506 (-5.0569, -1.3152) -> (-4.9868, -1.2577)
  line L507 (-4.9868, -1.2577) -> (-4.9194, -1.207)
  line L508 (-4.9194, -1.207) -> (-4.8581, -1.1647)
  line L509 (-4.8581, -1.1647) -> (-4.8009, -1.1288)
  line L510 (-4.8009, -1.1288) -> (-4.75, -1.0997)
  line L511 (-4.75, -1.0997) -> (-4.7061, -1.0769)
  line L512 (-4.7061, -1.0769) -> (-4.6364, -1.046)
  line L513 (-4.6364, -1.046) -> (-4.5924, -1.0307)
  line L514 (-4.5924, -1.0307) -> (-4.5075, -1.0081)
  line L515 (-4.5075, -1.0081) -> (-4.4514, -0.9867)
  line L516 (-4.4514, -0.9867) -> (-4.427, -0.9751)
  line L517 (-4.427, -0.9751) -> (-4.4051, -0.9628)
  line L518 (-4.4051, -0.9628) -> (-4.3856, -0.9502)
  line L519 (-4.3856, -0.9502) -> (-4.3686, -0.9372)
  line L520 (-4.3686, -0.9372) -> (-4.354, -0.9239)
  line L521 (-4.354, -0.9239) -> (-4.3419, -0.9105)
  line L522 (-4.3419, -0.9105) -> (-4.3323, -0.897)
  line L523 (-4.3323, -0.897) -> (-4.3252, -0.8836)
  line L524 (-4.3252, -0.8836) -> (-4.3205, -0.8703)
  line L525 (-4.3205, -0.8703) -> (-4.3182, -0.8572)
  line L526 (-4.3182, -0.8572) -> (-4.3194, -0.8383)
  line L527 (-4.3194, -0.8383) -> (-4.3458, -0.6883)
  line L528 (-4.3458, -0.6883) -> (-4.3671, -0.5375)
  line L529 (-4.3671, -0.5375) -> (-4.3718, -0.5191)
  line L530 (-4.3718, -0.5191) -> (-4.378, -0.5074)
  line L531 (-4.378, -0.5074) -> (-4.3865, -0.4962)
  line L532 (-4.3865, -0.4962) -> (-4.3975, -0.4856)
  line L533 (-4.3975, -0.4856) -> (-4.4108, -0.4758)
  line L534 (-4.4108, -0.4758) -> (-4.4264, -0.4668)
  line L535 (-4.4264, -0.4668) -> (-4.4444, -0.4587)
  line L536 (-4.4444, -0.4587) -> (-4.4646, -0.4516)
  line L537 (-4.4646, -0.4516) -> (-4.487, -0.4455)
  line L538 (-4.487, -0.4455) -> (-4.5117, -0.4407)
  line L539 (-4.5117, -0.4407) -> (-4.5385, -0.4371)
  line L540 (-4.5385, -0.4371) -> (-4.5984, -0.4341)
  line L541 (-4.5984, -0.4341) -> (-4.6862, -0.4388)
  line L542 (-4.6862, -0.4388) -> (-4.7327, -0.438)
  line L543 (-4.7327, -0.438) -> (-4.8085, -0.43)
  line L544 (-4.8085, -0.43) -> (-4.8574, -0.422)
  line L545 (-4.8574, -0.422) -> (-4.9147, -0.41)
  line L546 (-4.9147, -0.41) -> (-4.9802, -0.3935)
  line L547 (-4.9802, -0.3935) -> (-5.0516, -0.3723)
  line L548 (-5.0516, -0.3723) -> (-5.1313, -0.3449)
  line L549 (-5.1313, -0.3449) -> (-5.2159, -0.3118)
  line L550 (-5.2159, -0.3118) -> (-5.3081, -0.2712)
  line L551 (-5.3081, -0.2712) -> (-5.4053, -0.2235)
  line L552 (-5.4053, -0.2235) -> (-5.4973, -0.1736)
  arc A12 (-5.4973, 0.1736) -> (-5.4973, -0.1736) centre (0, 0) ccw
  line L553 (-5.4973, 0.1736) -> (-5.4053, 0.2235)
  line L554 (-5.4053, 0.2235) -> (-5.3081, 0.2712)
  line L555 (-5.3081, 0.2712) -> (-5.2159, 0.3118)
  line L556 (-5.2159, 0.3118) -> (-5.1313, 0.3449)
  line L557 (-5.1313, 0.3449) -> (-5.0516, 0.3723)
  line L558 (-5.0516, 0.3723) -> (-4.9802, 0.3935)
  line L559 (-4.9802, 0.3935) -> (-4.9147, 0.41)
  line L560 (-4.9147, 0.41) -> (-4.8574, 0.422)
  line L561 (-4.8574, 0.422) -> (-4.8085, 0.43)
  line L562 (-4.8085, 0.43) -> (-4.7327, 0.438)
  line L563 (-4.7327, 0.438) -> (-4.6862, 0.4388)
  line L564 (-4.6862, 0.4388) -> (-4.5984, 0.4341)
  line L565 (-4.5984, 0.4341) -> (-4.5385, 0.4371)
  line L566 (-4.5385, 0.4371) -> (-4.5117, 0.4407)
  line L567 (-4.5117, 0.4407) -> (-4.487, 0.4455)
  line L568 (-4.487, 0.4455) -> (-4.4646, 0.4516)
  line L569 (-4.4646, 0.4516) -> (-4.4444, 0.4587)
  line L570 (-4.4444, 0.4587) -> (-4.4264, 0.4668)
  line L571 (-4.4264, 0.4668) -> (-4.4108, 0.4758)
  line L572 (-4.4108, 0.4758) -> (-4.3975, 0.4856)
  line L573 (-4.3975, 0.4856) -> (-4.3865, 0.4962)
  line L574 (-4.3865, 0.4962) -> (-4.378, 0.5074)
  line L575 (-4.378, 0.5074) -> (-4.3718, 0.5191)
  line L576 (-4.3718, 0.5191) -> (-4.3671, 0.5375)
  line L577 (-4.3671, 0.5375) -> (-4.3458, 0.6883)
  line L578 (-4.3458, 0.6883) -> (-4.3194, 0.8383)
  line L579 (-4.3194, 0.8383) -> (-4.3182, 0.8572)
  line L580 (-4.3182, 0.8572) -> (-4.3205, 0.8703)
  line L581 (-4.3205, 0.8703) -> (-4.3252, 0.8836)
  line L582 (-4.3252, 0.8836) -> (-4.3323, 0.897)
  line L583 (-4.3323, 0.897) -> (-4.3419, 0.9105)
  line L584 (-4.3419, 0.9105) -> (-4.354, 0.9239)
  line L585 (-4.354, 0.9239) -> (-4.3686, 0.9372)
  line L586 (-4.3686, 0.9372) -> (-4.3856, 0.9502)
  line L587 (-4.3856, 0.9502) -> (-4.4051, 0.9628)
  line L588 (-4.4051, 0.9628) -> (-4.427, 0.9751)
  line L589 (-4.427, 0.9751) -> (-4.4514, 0.9867)
  line L590 (-4.4514, 0.9867) -> (-4.5075, 1.0081)
  line L591 (-4.5075, 1.0081) -> (-4.5924, 1.0307)
  line L592 (-4.5924, 1.0307) -> (-4.6364, 1.046)
  line L593 (-4.6364, 1.046) -> (-4.7061, 1.0769)
  line L594 (-4.7061, 1.0769) -> (-4.75, 1.0997)
  line L595 (-4.75, 1.0997) -> (-4.8009, 1.1288)
  line L596 (-4.8009, 1.1288) -> (-4.8581, 1.1647)
  line L597 (-4.8581, 1.1647) -> (-4.9194, 1.207)
  line L598 (-4.9194, 1.207) -> (-4.9868, 1.2577)
  line L599 (-4.9868, 1.2577) -> (-5.0569, 1.3152)
  line L600 (-5.0569, 1.3152) -> (-5.1322, 1.3823)
  line L601 (-5.1322, 1.3823) -> (-5.2098, 1.4578)
  line L602 (-5.2098, 1.4578) -> (-5.2818, 1.5336)
  arc A13 (-5.1745, 1.8639) -> (-5.2818, 1.5336) centre (0, 0) ccw
  line L603 (-5.1745, 1.8639) -> (-5.0717, 1.8829)
  line L604 (-5.0717, 1.8829) -> (-4.9645, 1.8983)
  line L605 (-4.9645, 1.8983) -> (-4.8642, 1.9084)
  line L606 (-4.8642, 1.9084) -> (-4.7736, 1.9137)
  line L607 (-4.7736, 1.9137) -> (-4.6893, 1.9151)
  line L608 (-4.6893, 1.9151) -> (-4.6149, 1.9132)
  line L609 (-4.6149, 1.9132) -> (-4.5475, 1.9087)
  line L610 (-4.5475, 1.9087) -> (-4.4892, 1.9023)
  line L611 (-4.4892, 1.9023) -> (-4.4403, 1.8949)
  line L612 (-4.4403, 1.8949) -> (-4.3657, 1.879)
  line L613 (-4.3657, 1.879) -> (-4.3212, 1.8655)
  line L614 (-4.3212, 1.8655) -> (-4.2391, 1.8339)
  line L615 (-4.2391, 1.8339) -> (-4.1813, 1.8182)
  line L616 (-4.1813, 1.8182) -> (-4.1547, 1.8133)
  line L617 (-4.1547, 1.8133) -> (-4.1297, 1.8103)
  line L618 (-4.1297, 1.8103) -> (-4.1065, 1.8091)
  line L619 (-4.1065, 1.8091) -> (-4.0851, 1.8096)
  line L620 (-4.0851, 1.8096) -> (-4.0655, 1.8118)
  line L621 (-4.0655, 1.8118) -> (-4.0479, 1.8155)
  line L622 (-4.0479, 1.8155) -> (-4.0322, 1.8208)
  line L623 (-4.0322, 1.8208) -> (-4.0185, 1.8274)
  line L624 (-4.0185, 1.8274) -> (-4.0069, 1.8354)
  line L625 (-4.0069, 1.8354) -> (-3.9974, 1.8447)
  line L626 (-3.9974, 1.8447) -> (-3.9872, 1.8607)
  line L627 (-3.9872, 1.8607) -> (-3.9204, 1.9976)
  line L628 (-3.9204, 1.9976) -> (-3.8489, 2.1321)
  line L629 (-3.8489, 2.1321) -> (-3.842, 2.1497)
  line L630 (-3.842, 2.1497) -> (-3.8401, 2.1628)
  line L631 (-3.8401, 2.1628) -> (-3.8404, 2.1769)
  line L632 (-3.8404, 2.1769) -> (-3.8431, 2.1919)
  line L633 (-3.8431, 2.1919) -> (-3.8481, 2.2077)
  line L634 (-3.8481, 2.2077) -> (-3.8554, 2.2242)
  line L635 (-3.8554, 2.2242) -> (-3.8652, 2.2413)
  line L636 (-3.8652, 2.2413) -> (-3.8773, 2.2589)
  line L637 (-3.8773, 2.2589) -> (-3.892, 2.277)
  line L638 (-3.892, 2.277) -> (-3.9091, 2.2954)
  line L639 (-3.9091, 2.2954) -> (-3.9286, 2.314)
  line L640 (-3.9286, 2.314) -> (-3.9753, 2.3516)
  line L641 (-3.9753, 2.3516) -> (-4.0491, 2.3994)
  line L642 (-4.0491, 2.3994) -> (-4.0862, 2.4275)
  line L643 (-4.0862, 2.4275) -> (-4.1429, 2.4785)
  line L644 (-4.1429, 2.4785) -> (-4.1777, 2.5137)
  line L645 (-4.1777, 2.5137) -> (-4.2171, 2.5571)
  line L646 (-4.2171, 2.5571) -> (-4.2604, 2.609)
  line L647 (-4.2604, 2.609) -> (-4.3057, 2.6681)
  line L648 (-4.3057, 2.6681) -> (-4.3541, 2.7371)
  line L649 (-4.3541, 2.7371) -> (-4.403, 2.8135)
  line L650 (-4.403, 2.8135) -> (-4.4538, 2.9006)
  line L651 (-4.4538, 2.9006) -> (-4.5044, 2.9964)
  line L652 (-4.5044, 2.9964) -> (-4.5494, 3.0907)
  arc A14 (-4.3453, 3.3717) -> (-4.5494, 3.0907) centre (0, 0) ccw
  line L653 (-4.3453, 3.3717) -> (-4.2416, 3.358)
  line L654 (-4.2416, 3.358) -> (-4.1349, 3.3395)
  line L655 (-4.1349, 3.3395) -> (-4.0364, 3.3181)
  line L656 (-4.0364, 3.3181) -> (-3.9486, 3.2952)
  line L657 (-3.9486, 3.2952) -> (-3.868, 3.2704)
  line L658 (-3.868, 3.2704) -> (-3.7978, 3.2457)
  line L659 (-3.7978, 3.2457) -> (-3.7351, 3.2205)
  line L660 (-3.7351, 3.2205) -> (-3.6817, 3.1965)
  line L661 (-3.6817, 3.1965) -> (-3.6374, 3.1743)
  line L662 (-3.6374, 3.1743) -> (-3.5714, 3.1361)
  line L663 (-3.5714, 3.1361) -> (-3.5332, 3.1095)
  line L664 (-3.5332, 3.1095) -> (-3.465, 3.0541)
  line L665 (-3.465, 3.0541) -> (-3.4148, 3.0213)
  line L666 (-3.4148, 3.0213) -> (-3.391, 3.0084)
  line L667 (-3.391, 3.0084) -> (-3.3682, 2.9979)
  line L668 (-3.3682, 2.9979) -> (-3.3465, 2.9895)
  line L669 (-3.3465, 2.9895) -> (-3.326, 2.9834)
  line L670 (-3.326, 2.9834) -> (-3.3067, 2.9794)
  line L671 (-3.3067, 2.9794) -> (-3.2887, 2.9775)
  line L672 (-3.2887, 2.9775) -> (-3.2722, 2.9777)
  line L673 (-3.2722, 2.9777) -> (-3.2571, 2.9798)
  line L674 (-3.2571, 2.9798) -> (-3.2436, 2.9838)
  line L675 (-3.2436, 2.9838) -> (-3.2317, 2.9896)
  line L676 (-3.2317, 2.9896) -> (-3.2171, 3.0017)
  line L677 (-3.2171, 3.0017) -> (-3.1113, 3.1113)
  line L678 (-3.1113, 3.1113) -> (-3.0017, 3.2171)
  line L679 (-3.0017, 3.2171) -> (-2.9896, 3.2317)
  line L680 (-2.9896, 3.2317) -> (-2.9838, 3.2436)
  line L681 (-2.9838, 3.2436) -> (-2.9798, 3.2571)
  line L682 (-2.9798, 3.2571) -> (-2.9777, 3.2722)
  line L683 (-2.9777, 3.2722) -> (-2.9775, 3.2887)
  line L684 (-2.9775, 3.2887) -> (-2.9794, 3.3067)
  line L685 (-2.9794, 3.3067) -> (-2.9834, 3.326)
  line L686 (-2.9834, 3.326) -> (-2.9895, 3.3465)
  line L687 (-2.9895, 3.3465) -> (-2.9979, 3.3682)
  line L688 (-2.9979, 3.3682) -> (-3.0084, 3.391)
  line L689 (-3.0084, 3.391) -> (-3.0213, 3.4148)
  line L690 (-3.0213, 3.4148) -> (-3.0541, 3.465)
  line L691 (-3.0541, 3.465) -> (-3.1095, 3.5332)
  line L692 (-3.1095, 3.5332) -> (-3.1361, 3.5714)
  line L693 (-3.1361, 3.5714) -> (-3.1743, 3.6374)
  line L694 (-3.1743, 3.6374) -> (-3.1965, 3.6817)
  line L695 (-3.1965, 3.6817) -> (-3.2205, 3.7351)
  line L696 (-3.2205, 3.7351) -> (-3.2457, 3.7978)
  line L697 (-3.2457, 3.7978) -> (-3.2704, 3.868)
  line L698 (-3.2704, 3.868) -> (-3.2952, 3.9486)
  line L699 (-3.2952, 3.9486) -> (-3.3181, 4.0364)
  line L700 (-3.3181, 4.0364) -> (-3.3395, 4.1349)
  line L701 (-3.3395, 4.1349) -> (-3.358, 4.2416)
  line L702 (-3.358, 4.2416) -> (-3.3717, 4.3453)
  arc A15 (-3.0907, 4.5494) -> (-3.3717, 4.3453) centre (0, 0) ccw
  line L703 (-3.0907, 4.5494) -> (-2.9964, 4.5044)
  line L704 (-2.9964, 4.5044) -> (-2.9006, 4.4538)
  line L705 (-2.9006, 4.4538) -> (-2.8135, 4.403)
  line L706 (-2.8135, 4.403) -> (-2.7371, 4.3541)
  line L707 (-2.7371, 4.3541) -> (-2.6681, 4.3057)
  line L708 (-2.6681, 4.3057) -> (-2.609, 4.2604)
  line L709 (-2.609, 4.2604) -> (-2.5571, 4.2171)
  line L710 (-2.5571, 4.2171) -> (-2.5137, 4.1777)
  line L711 (-2.5137, 4.1777) -> (-2.4785, 4.1429)
  line L712 (-2.4785, 4.1429) -> (-2.4275, 4.0862)
  line L713 (-2.4275, 4.0862) -> (-2.3994, 4.0491)
  line L714 (-2.3994, 4.0491) -> (-2.3516, 3.9753)
  line L715 (-2.3516, 3.9753) -> (-2.314, 3.9286)
  line L716 (-2.314, 3.9286) -> (-2.2954, 3.9091)
  line L717 (-2.2954, 3.9091) -> (-2.277, 3.892)
  line L718 (-2.277, 3.892) -> (-2.2589, 3.8773)
  line L719 (-2.2589, 3.8773) -> (-2.2413, 3.8652)
  line L720 (-2.2413, 3.8652) -> (-2.2242, 3.8554)
  line L721 (-2.2242, 3.8554) -> (-2.2077, 3.8481)
  line L722 (-2.2077, 3.8481) -> (-2.1919, 3.8431)
  line L723 (-2.1919, 3.8431) -> (-2.1769, 3.8404)
  line L724 (-2.1769, 3.8404) -> (-2.1628, 3.8401)
  line L725 (-2.1628, 3.8401) -> (-2.1497, 3.842)
  line L726 (-2.1497, 3.842) -> (-2.1321, 3.8489)
  line L727 (-2.1321, 3.8489) -> (-1.9976, 3.9204)
  line L728 (-1.9976, 3.9204) -> (-1.8607, 3.9872)
  line L729 (-1.8607, 3.9872) -> (-1.8447, 3.9974)
  line L730 (-1.8447, 3.9974) -> (-1.8354, 4.0069)
  line L731 (-1.8354, 4.0069) -> (-1.8274, 4.0185)
  line L732 (-1.8274, 4.0185) -> (-1.8208, 4.0322)
  line L733 (-1.8208, 4.0322) -> (-1.8155, 4.0479)
  line L734 (-1.8155, 4.0479) -> (-1.8118, 4.0655)
  line L735 (-1.8118, 4.0655) -> (-1.8096, 4.0851)
  line L736 (-1.8096, 4.0851) -> (-1.8091, 4.1065)
  line L737 (-1.8091, 4.1065) -> (-1.8103, 4.1297)
  line L738 (-1.8103, 4.1297) -> (-1.8133, 4.1547)
  line L739 (-1.8133, 4.1547) -> (-1.8182, 4.1813)
  line L740 (-1.8182, 4.1813) -> (-1.8339, 4.2391)
  line L741 (-1.8339, 4.2391) -> (-1.8655, 4.3212)
  line L742 (-1.8655, 4.3212) -> (-1.879, 4.3657)
  line L743 (-1.879, 4.3657) -> (-1.8949, 4.4403)
  line L744 (-1.8949, 4.4403) -> (-1.9023, 4.4892)
  line L745 (-1.9023, 4.4892) -> (-1.9087, 4.5475)
  line L746 (-1.9087, 4.5475) -> (-1.9132, 4.6149)
  line L747 (-1.9132, 4.6149) -> (-1.9151, 4.6893)
  line L748 (-1.9151, 4.6893) -> (-1.9137, 4.7736)
  line L749 (-1.9137, 4.7736) -> (-1.9084, 4.8642)
  line L750 (-1.9084, 4.8642) -> (-1.8983, 4.9645)
  line L751 (-1.8983, 4.9645) -> (-1.8829, 5.0717)
  line L752 (-1.8829, 5.0717) -> (-1.8639, 5.1745)
  arc A16 (-1.5336, 5.2818) -> (-1.8639, 5.1745) centre (0, 0) ccw
  line L753 (-1.5336, 5.2818) -> (-1.4578, 5.2098)
  line L754 (-1.4578, 5.2098) -> (-1.3823, 5.1322)
  line L755 (-1.3823, 5.1322) -> (-1.3152, 5.0569)
  line L756 (-1.3152, 5.0569) -> (-1.2577, 4.9868)
  line L757 (-1.2577, 4.9868) -> (-1.207, 4.9194)
  line L758 (-1.207, 4.9194) -> (-1.1647, 4.8581)
  line L759 (-1.1647, 4.8581) -> (-1.1288, 4.8009)
  line L760 (-1.1288, 4.8009) -> (-1.0997, 4.75)
  line L761 (-1.0997, 4.75) -> (-1.0769, 4.7061)
  line L762 (-1.0769, 4.7061) -> (-1.046, 4.6364)
  line L763 (-1.046, 4.6364) -> (-1.0307, 4.5924)
  line L764 (-1.0307, 4.5924) -> (-1.0081, 4.5075)
  line L765 (-1.0081, 4.5075) -> (-0.9867, 4.4514)
  line L766 (-0.9867, 4.4514) -> (-0.9751, 4.427)
  line L767 (-0.9751, 4.427) -> (-0.9628, 4.4051)
  line L768 (-0.9628, 4.4051) -> (-0.9502, 4.3856)
  line L769 (-0.9502, 4.3856) -> (-0.9372, 4.3686)
  line L770 (-0.9372, 4.3686) -> (-0.9239, 4.354)
  line L771 (-0.9239, 4.354) -> (-0.9105, 4.3419)
  line L772 (-0.9105, 4.3419) -> (-0.897, 4.3323)
  line L773 (-0.897, 4.3323) -> (-0.8836, 4.3252)
  line L774 (-0.8836, 4.3252) -> (-0.8703, 4.3205)
  line L775 (-0.8703, 4.3205) -> (-0.8572, 4.3182)
  line L776 (-0.8572, 4.3182) -> (-0.8383, 4.3194)
  line L777 (-0.8383, 4.3194) -> (-0.6883, 4.3458)
  line L778 (-0.6883, 4.3458) -> (-0.5375, 4.3671)
  line L779 (-0.5375, 4.3671) -> (-0.5191, 4.3718)
  line L780 (-0.5191, 4.3718) -> (-0.5074, 4.378)
  line L781 (-0.5074, 4.378) -> (-0.4962, 4.3865)
  line L782 (-0.4962, 4.3865) -> (-0.4856, 4.3975)
  line L783 (-0.4856, 4.3975) -> (-0.4758, 4.4108)
  line L784 (-0.4758, 4.4108) -> (-0.4668, 4.4264)
  line L785 (-0.4668, 4.4264) -> (-0.4587, 4.4444)
  line L786 (-0.4587, 4.4444) -> (-0.4516, 4.4646)
  line L787 (-0.4516, 4.4646) -> (-0.4455, 4.487)
  line L788 (-0.4455, 4.487) -> (-0.4407, 4.5117)
  line L789 (-0.4407, 4.5117) -> (-0.4371, 4.5385)
  line L790 (-0.4371, 4.5385) -> (-0.4341, 4.5984)
  line L791 (-0.4341, 4.5984) -> (-0.4388, 4.6862)
  line L792 (-0.4388, 4.6862) -> (-0.438, 4.7327)
  line L793 (-0.438, 4.7327) -> (-0.43, 4.8085)
  line L794 (-0.43, 4.8085) -> (-0.422, 4.8574)
  line L795 (-0.422, 4.8574) -> (-0.41, 4.9147)
  line L796 (-0.41, 4.9147) -> (-0.3935, 4.9802)
  line L797 (-0.3935, 4.9802) -> (-0.3723, 5.0516)
  line L798 (-0.3723, 5.0516) -> (-0.3449, 5.1313)
  line L799 (-0.3449, 5.1313) -> (-0.3118, 5.2159)
  line L800 (-0.3118, 5.2159) -> (-0.2712, 5.3081)
  line L801 (-0.2712, 5.3081) -> (-0.2235, 5.4053)
  line L802 (-0.2235, 5.4053) -> (-0.1736, 5.4973)
  arc A17 (0.1736, 5.4973) -> (-0.1736, 5.4973) centre (0, 0) ccw
  line L803 (0.1736, 5.4973) -> (0.2235, 5.4053)
  line L804 (0.2235, 5.4053) -> (0.2712, 5.3081)
  line L805 (0.2712, 5.3081) -> (0.3118, 5.2159)
  line L806 (0.3118, 5.2159) -> (0.3449, 5.1313)
  line L807 (0.3449, 5.1313) -> (0.3723, 5.0516)
  line L808 (0.3723, 5.0516) -> (0.3935, 4.9802)
  line L809 (0.3935, 4.9802) -> (0.41, 4.9147)
  line L810 (0.41, 4.9147) -> (0.422, 4.8574)
  line L811 (0.422, 4.8574) -> (0.43, 4.8085)
  line L812 (0.43, 4.8085) -> (0.438, 4.7327)
  line L813 (0.438, 4.7327) -> (0.4388, 4.6862)
  line L814 (0.4388, 4.6862) -> (0.4341, 4.5984)
  line L815 (0.4341, 4.5984) -> (0.4371, 4.5385)
  line L816 (0.4371, 4.5385) -> (0.4407, 4.5117)
  line L817 (0.4407, 4.5117) -> (0.4455, 4.487)
  line L818 (0.4455, 4.487) -> (0.4516, 4.4646)
  line L819 (0.4516, 4.4646) -> (0.4587, 4.4444)
  line L820 (0.4587, 4.4444) -> (0.4668, 4.4264)
  line L821 (0.4668, 4.4264) -> (0.4758, 4.4108)
  line L822 (0.4758, 4.4108) -> (0.4856, 4.3975)
  line L823 (0.4856, 4.3975) -> (0.4962, 4.3865)
  line L824 (0.4962, 4.3865) -> (0.5074, 4.378)
  line L825 (0.5074, 4.378) -> (0.5191, 4.3718)
  line L826 (0.5191, 4.3718) -> (0.5375, 4.3671)
  line L827 (0.5375, 4.3671) -> (0.6883, 4.3458)
  line L828 (0.6883, 4.3458) -> (0.8383, 4.3194)
  line L829 (0.8383, 4.3194) -> (0.8572, 4.3182)
  line L830 (0.8572, 4.3182) -> (0.8703, 4.3205)
  line L831 (0.8703, 4.3205) -> (0.8836, 4.3252)
  line L832 (0.8836, 4.3252) -> (0.897, 4.3323)
  line L833 (0.897, 4.3323) -> (0.9105, 4.3419)
  line L834 (0.9105, 4.3419) -> (0.9239, 4.354)
  line L835 (0.9239, 4.354) -> (0.9372, 4.3686)
  line L836 (0.9372, 4.3686) -> (0.9502, 4.3856)
  line L837 (0.9502, 4.3856) -> (0.9628, 4.4051)
  line L838 (0.9628, 4.4051) -> (0.9751, 4.427)
  line L839 (0.9751, 4.427) -> (0.9867, 4.4514)
  line L840 (0.9867, 4.4514) -> (1.0081, 4.5075)
  line L841 (1.0081, 4.5075) -> (1.0307, 4.5924)
  line L842 (1.0307, 4.5924) -> (1.046, 4.6364)
  line L843 (1.046, 4.6364) -> (1.0769, 4.7061)
  line L844 (1.0769, 4.7061) -> (1.0997, 4.75)
  line L845 (1.0997, 4.75) -> (1.1288, 4.8009)
  line L846 (1.1288, 4.8009) -> (1.1647, 4.8581)
  line L847 (1.1647, 4.8581) -> (1.207, 4.9194)
  line L848 (1.207, 4.9194) -> (1.2577, 4.9868)
  line L849 (1.2577, 4.9868) -> (1.3152, 5.0569)
  line L850 (1.3152, 5.0569) -> (1.3823, 5.1322)
  line L851 (1.3823, 5.1322) -> (1.4578, 5.2098)
  line L852 (1.4578, 5.2098) -> (1.5336, 5.2818)
  arc A18 (1.8639, 5.1745) -> (1.5336, 5.2818) centre (0, 0) ccw
  line L853 (1.8639, 5.1745) -> (1.8829, 5.0717)
  line L854 (1.8829, 5.0717) -> (1.8983, 4.9645)
  line L855 (1.8983, 4.9645) -> (1.9084, 4.8642)
  line L856 (1.9084, 4.8642) -> (1.9137, 4.7736)
  line L857 (1.9137, 4.7736) -> (1.9151, 4.6893)
  line L858 (1.9151, 4.6893) -> (1.9132, 4.6149)
  line L859 (1.9132, 4.6149) -> (1.9087, 4.5475)
  line L860 (1.9087, 4.5475) -> (1.9023, 4.4892)
  line L861 (1.9023, 4.4892) -> (1.8949, 4.4403)
  line L862 (1.8949, 4.4403) -> (1.879, 4.3657)
  line L863 (1.879, 4.3657) -> (1.8655, 4.3212)
  line L864 (1.8655, 4.3212) -> (1.8339, 4.2391)
  line L865 (1.8339, 4.2391) -> (1.8182, 4.1813)
  line L866 (1.8182, 4.1813) -> (1.8133, 4.1547)
  line L867 (1.8133, 4.1547) -> (1.8103, 4.1297)
  line L868 (1.8103, 4.1297) -> (1.8091, 4.1065)
  line L869 (1.8091, 4.1065) -> (1.8096, 4.0851)
  line L870 (1.8096, 4.0851) -> (1.8118, 4.0655)
  line L871 (1.8118, 4.0655) -> (1.8155, 4.0479)
  line L872 (1.8155, 4.0479) -> (1.8208, 4.0322)
  line L873 (1.8208, 4.0322) -> (1.8274, 4.0185)
  line L874 (1.8274, 4.0185) -> (1.8354, 4.0069)
  line L875 (1.8354, 4.0069) -> (1.8447, 3.9974)
  line L876 (1.8447, 3.9974) -> (1.8607, 3.9872)
  line L877 (1.8607, 3.9872) -> (1.9976, 3.9204)
  line L878 (1.9976, 3.9204) -> (2.1321, 3.8489)
  line L879 (2.1321, 3.8489) -> (2.1497, 3.842)
  line L880 (2.1497, 3.842) -> (2.1628, 3.8401)
  line L881 (2.1628, 3.8401) -> (2.1769, 3.8404)
  line L882 (2.1769, 3.8404) -> (2.1919, 3.8431)
  line L883 (2.1919, 3.8431) -> (2.2077, 3.8481)
  line L884 (2.2077, 3.8481) -> (2.2242, 3.8554)
  line L885 (2.2242, 3.8554) -> (2.2413, 3.8652)
  line L886 (2.2413, 3.8652) -> (2.2589, 3.8773)
  line L887 (2.2589, 3.8773) -> (2.277, 3.892)
  line L888 (2.277, 3.892) -> (2.2954, 3.9091)
  line L889 (2.2954, 3.9091) -> (2.314, 3.9286)
  line L890 (2.314, 3.9286) -> (2.3516, 3.9753)
  line L891 (2.3516, 3.9753) -> (2.3994, 4.0491)
  line L892 (2.3994, 4.0491) -> (2.4275, 4.0862)
  line L893 (2.4275, 4.0862) -> (2.4785, 4.1429)
  line L894 (2.4785, 4.1429) -> (2.5137, 4.1777)
  line L895 (2.5137, 4.1777) -> (2.5571, 4.2171)
  line L896 (2.5571, 4.2171) -> (2.609, 4.2604)
  line L897 (2.609, 4.2604) -> (2.6681, 4.3057)
  line L898 (2.6681, 4.3057) -> (2.7371, 4.3541)
  line L899 (2.7371, 4.3541) -> (2.8135, 4.403)
  line L900 (2.8135, 4.403) -> (2.9006, 4.4538)
  line L901 (2.9006, 4.4538) -> (2.9964, 4.5044)
  line L902 (2.9964, 4.5044) -> (3.0907, 4.5494)
  arc A19 (3.3717, 4.3453) -> (3.0907, 4.5494) centre (0, 0) ccw
  line L903 (3.3717, 4.3453) -> (3.358, 4.2416)
  line L904 (3.358, 4.2416) -> (3.3395, 4.1349)
  line L905 (3.3395, 4.1349) -> (3.3181, 4.0364)
  line L906 (3.3181, 4.0364) -> (3.2952, 3.9486)
  line L907 (3.2952, 3.9486) -> (3.2704, 3.868)
  line L908 (3.2704, 3.868) -> (3.2457, 3.7978)
  line L909 (3.2457, 3.7978) -> (3.2205, 3.7351)
  line L910 (3.2205, 3.7351) -> (3.1965, 3.6817)
  line L911 (3.1965, 3.6817) -> (3.1743, 3.6374)
  line L912 (3.1743, 3.6374) -> (3.1361, 3.5714)
  line L913 (3.1361, 3.5714) -> (3.1095, 3.5332)
  line L914 (3.1095, 3.5332) -> (3.0541, 3.465)
  line L915 (3.0541, 3.465) -> (3.0213, 3.4148)
  line L916 (3.0213, 3.4148) -> (3.0084, 3.391)
  line L917 (3.0084, 3.391) -> (2.9979, 3.3682)
  line L918 (2.9979, 3.3682) -> (2.9895, 3.3465)
  line L919 (2.9895, 3.3465) -> (2.9834, 3.326)
  line L920 (2.9834, 3.326) -> (2.9794, 3.3067)
  line L921 (2.9794, 3.3067) -> (2.9775, 3.2887)
  line L922 (2.9775, 3.2887) -> (2.9777, 3.2722)
  line L923 (2.9777, 3.2722) -> (2.9798, 3.2571)
  line L924 (2.9798, 3.2571) -> (2.9838, 3.2436)
  line L925 (2.9838, 3.2436) -> (2.9896, 3.2317)
  line L926 (2.9896, 3.2317) -> (3.0017, 3.2171)
  line L927 (3.0017, 3.2171) -> (3.1113, 3.1113)
  line L928 (3.1113, 3.1113) -> (3.2171, 3.0017)
  line L929 (3.2171, 3.0017) -> (3.2317, 2.9896)
  line L930 (3.2317, 2.9896) -> (3.2436, 2.9838)
  line L931 (3.2436, 2.9838) -> (3.2571, 2.9798)
  line L932 (3.2571, 2.9798) -> (3.2722, 2.9777)
  line L933 (3.2722, 2.9777) -> (3.2887, 2.9775)
  line L934 (3.2887, 2.9775) -> (3.3067, 2.9794)
  line L935 (3.3067, 2.9794) -> (3.326, 2.9834)
  line L936 (3.326, 2.9834) -> (3.3465, 2.9895)
  line L937 (3.3465, 2.9895) -> (3.3682, 2.9979)
  line L938 (3.3682, 2.9979) -> (3.391, 3.0084)
  line L939 (3.391, 3.0084) -> (3.4148, 3.0213)
  line L940 (3.4148, 3.0213) -> (3.465, 3.0541)
  line L941 (3.465, 3.0541) -> (3.5332, 3.1095)
  line L942 (3.5332, 3.1095) -> (3.5714, 3.1361)
  line L943 (3.5714, 3.1361) -> (3.6374, 3.1743)
  line L944 (3.6374, 3.1743) -> (3.6817, 3.1965)
  line L945 (3.6817, 3.1965) -> (3.7351, 3.2205)
  line L946 (3.7351, 3.2205) -> (3.7978, 3.2457)
  line L947 (3.7978, 3.2457) -> (3.868, 3.2704)
  line L948 (3.868, 3.2704) -> (3.9486, 3.2952)
  line L949 (3.9486, 3.2952) -> (4.0364, 3.3181)
  line L950 (4.0364, 3.3181) -> (4.1349, 3.3395)
  line L951 (4.1349, 3.3395) -> (4.2416, 3.358)